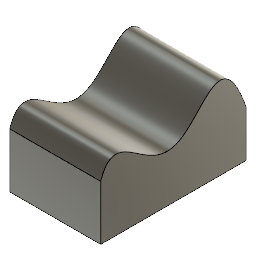
6.7 silhouette split (Autodesk Fusion 360 design; units mm, degrees)
Autodesk Fusion 360 part; units mm, degrees
sketch "Sketch1" plane through (0, 0, 0) normal (1, 0, 0) x (0, 1, 0)
  spline S0 degree 5 poles (-51.5844, 15.0722) (-51.1338, 16.4427) (-50.1685, 18.9461) (-48.5283, 21.9883) (-45.9553, 24.6126) (-42.1, 25.5539) (-37.6337, 24.3549) (-32.6277, 21.4713) (-27.2098, 17.6899) (-21.539, 13.9438) (-15.7849, 11.1597) (-10.1046, 10.0861) (-4.6236, 11.1453) (0.5918, 14.2207) (5.5285, 18.7333) (10.2087, 23.8285) (14.6774, 28.5239) (18.9875, 31.8633) (23.1865, 33.0824) (27.3054, 31.7267) (31.3634, 27.554) (34.5691, 21.8904) (36.9521, 16.3321) (38.5314, 12.0464) (39.3187, 9.7585) knots 0 0 0 0 0 0 0.05 0.1 0.15 0.2 0.25 0.3 0.35 0.4 0.45 0.5 0.55 0.6 0.65 0.7 0.75 0.8 0.85 0.9 0.95 1 1 1 1 1 1
  line L0 (-51.5844, 15.0722) -> (-51.5844, -19.0876)
  line L1 (-51.5844, -19.0876) -> (39.3187, -19.0876)
  line L2 (39.3187, -19.0876) -> (39.3187, 9.7585)
  point P0 (-38.1103, 24.1815)
  point P1 (-8.5051, 10.7073)
  point P2 (18.0637, 30.8237)
  constraint vertical L0
  constraint perpendicular L0 L1
  constraint perpendicular L1 L2
extrude "Extrude1" add sketch "Sketch1" along normal blind 56.855
